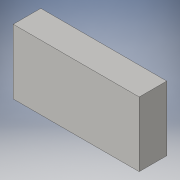
# Autodesk Inventor part: battery sumo jeffrey p
Saved by Autodesk Inventor 2016 (Build 200138000, 138)
## iProperties
Created: 2017-08-31
Part Number: battery sumo jeffrey p
Material: Generic
Document SubType Name: Modeling
Designer: student
Density: 1 g/cm^3
Appearance: Default
Author: student
Autodesk Inventor part; units mm, degrees
ref_plane "YZ Plane" through (0, 0, 0) normal (1, 0, 0) x (0, 1, 0)
ref_plane "XZ Plane" through (0, 0, 0) normal (0, 1, 0) x (-1, 0, 0)
ref_plane "XY Plane" through (0, 0, 0) normal (0, 0, 1) x (1, 0, 0)
sketch "Sketch1" plane through (0, 0, 0) normal (0, 0, 1) x (1, 0, 0)
  line L0 (-29.0068, -14.8971) -> (29.0068, -14.8971)
  line L1 (29.0068, -14.8971) -> (29.0068, 14.8971)
  line L2 (29.0068, 14.8971) -> (-29.0068, 14.8971)
  line L3 (-29.0068, 14.8971) -> (-29.0068, -14.8971)
  line L4 (-29.0068, -14.8971) -> (29.0068, 14.8971) construction
  line L5 (29.0068, -14.8971) -> (-29.0068, 14.8971) construction
  point P0 (0, 0)
  dimension "d0" = 29.7942
  dimension "d1" = 58.0136
  constraints: 12 end point, 2 midpoint, 2 parallel, 1 horizontal, 1 perpendicular
  measures "d0" distance between parallel lines of L0 L2
  measures "d1" distance between parallel lines of L1 L3
extrude "Extrusion1" add sketch "Sketch1" along normal blind 12.7
body "Solid1"
